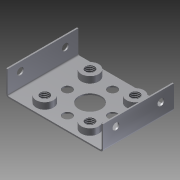
# Autodesk Inventor part: Servo Bracket
Saved by Autodesk Inventor 2012 (Build 160160000, 160)
## iProperties
Created: 2011-10-07
Part Number: Servo Bracket
Material: Default
Document SubType Name: Sheet Metal
Designer: KuttaA
Density: 1 g/cm^3
Sheet Metal Rule: Default
Author: KuttaA
Autodesk Inventor part; units mm, degrees
ref_plane "YZ Plane" through (0, 0, 0) normal (1, 0, 0) x (0, 1, 0)
ref_plane "XZ Plane" through (0, 0, 0) normal (0, 1, 0) x (-1, 0, 0)
ref_plane "XY Plane" through (0, 0, 0) normal (0, 0, 1) x (1, 0, 0)
sketch "Sketch1" plane through (0, 0, 0) normal (0, 0, 1) x (1, 0, 0)
  line L0 (-17.23, 12.6) -> (17.23, 12.6)
  line L1 (17.23, 12.6) -> (17.23, -12.6)
  line L2 (17.23, -12.6) -> (-17.23, -12.6)
  line L3 (-17.23, -12.6) -> (-17.23, 12.6)
  point P0 (0, 0)
  dimension "d0" = 17.23
  dimension "d1" = 34.46
  dimension "d2" = 12.6
  dimension "d3" = 25.2
  measures "d0" distance from line of L1 point (0, 0)
  measures "d1" distance between parallel lines of L1 L3
  measures "d2" distance from line of L0 point (0, 0)
  measures "d3" distance of L2.end L0.start
extrude "Plate1" add sketch "Sketch1" along normal blind 0.5
sketch "Sketch4" plane through (-16.73, -12.6, 0) normal (-1, 0, 0) x (0, -1, 0)
  line L0 (-25.2, 0) -> (0, 0)
  line L1 (0, 0) -> (0, 8.75)
  line L2 (0, 8.75) -> (-25.2, 8.75)
  line L3 (-25.2, 8.75) -> (-25.2, 0)
  constraints: 4 end point, 4 other
edge flange "Flange1" height 8.75 angle 90 thickness 0.5 bend radius 0.5 thickness toward (-1, 0, 0) relief tear relief width 0.5 relief depth 0.25 edges at (-17.23, 0, 0.5) wall of the first edge with corners at (-16.73, 12.6, 0) (-16.73, -12.6, 0) (-16.73, -12.6, 8.75) (-16.73, 12.6, 8.75)
bend "Bend1"
corner "Corner1"
sketch "Sketch5" plane through (16.73, 12.6, 0) normal (1, 0, 0) x (0, 1, 0)
  line L0 (-25.2, 0) -> (0, 0)
  line L1 (0, 0) -> (0, 8.75)
  line L2 (0, 8.75) -> (-25.2, 8.75)
  line L3 (-25.2, 8.75) -> (-25.2, 0)
  constraints: 4 end point, 4 other
edge flange "Flange2" height 8.75 angle 90 thickness 0.5 bend radius 0.5 thickness toward (1, 0, 0) relief tear relief width 0.5 relief depth 0.25 edges at (17.23, 0, 0.5) wall of the first edge with corners at (16.73, -12.6, 0) (16.73, 12.6, 0) (16.73, 12.6, 8.75) (16.73, -12.6, 8.75)
bend "Bend2"
corner "Corner2"
sketch "Sketch6" plane through (0, 0, 0.5) normal (0, 0, 1) x (1, 0, 0)
  circle A0 centre (0, 0) radius 4
  circle A1 centre (0, 8.04) radius 1.65
  circle A2 centre (0, -8.04) radius 1.65
  circle A3 centre (8.04, 0) radius 1.65
  circle A4 centre (-8.04, 0) radius 1.65
  line L0 (16.23, -12.6) -> (-16.23, -12.6) projected
  line L1 (-16.23, 12.6) -> (16.23, 12.6) projected
  dimension "d26" = 3.3
  dimension "d27" = 8
  dimension "d29" = 4.56
  dimension "d30" = 4.56
  dimension "d31" = 8.04
  dimension "d32" = 8.04
  dimension "d33" = 8.04
  constraints: 5 centre point, 3 equal radius, 1 coincident
  measures "d26" diameter of A4
  measures "d27" diameter of A0
  measures "d29" distance from line of L0 A2.centre
  measures "d30" distance from line of A1.centre L1
  measures "d31" distance of point (0, 0) A1.centre
  measures "d32" distance of A3.centre point (0, 0)
  measures "d33" distance of A4.centre point (0, 0)
extrude "Extrusion1" cut sketch "Sketch6" against normal through all
sketch "Sketch7" plane through (0, 0, 0.5) normal (0, 0, 1) x (1, 0, 0)
  circle A0 centre (0, 8.04) radius 1.65 projected
  circle A1 centre (-8.04, 0) radius 1.65 projected
  circle A2 centre (-8.04, 8.04) radius 1.6
  line L0 (0, -17.64) -> (0, 17.64) projected
  line L1 (-24.122, 0) -> (24.122, 0) projected
  circle A3 centre (8.04, 8.04) radius 1.6
  circle A4 centre (-8.04, -8.04) radius 1.6
  circle A5 centre (8.04, -8.04) radius 1.6
  point P0 (0, 0)
  dimension "d36" = 3.2
  constraints: 4 centre point, 3 symmetric about line, 3 other
  measures "d36" diameter of A2
extrude "Extrusion2" cut sketch "Sketch7" against normal through all contours A2 | A3 | A4 | A5
sketch "Sketch8" plane through (0, 0, 0.5) normal (0, 0, 1) x (1, 0, 0)
  circle A0 centre (-8.04, 8.04) radius 1.6 projected
  circle A1 centre (8.04, 8.04) radius 1.6 projected
  circle A2 centre (8.04, -8.04) radius 1.6 projected
  circle A3 centre (-8.04, -8.04) radius 1.6 projected
  circle A4 centre (-8.04, 8.04) radius 3.1
  circle A5 centre (8.04, 8.04) radius 3.1
  circle A6 centre (8.04, -8.04) radius 3.1
  circle A7 centre (-8.04, -8.04) radius 3.1
  point P0 (0, 0)
  dimension "d39" = 6.2
  constraints: 4 centre point, 4 coincident, 3 equal radius
  measures "d39" diameter of A4
extrude "Extrusion3" add sketch "Sketch8" along normal blind 2.28
thread "Thread1" size "M3.5x0.6" class "6H" standard "ANSI Metric M Profile" full length
thread "Thread2" size "M3.5x0.6" class "6H" standard "ANSI Metric M Profile" full length
thread "Thread3" size "M3.5x0.6" class "6H" standard "ANSI Metric M Profile" full length
thread "Thread4" size "M3.5x0.6" class "6H" standard "ANSI Metric M Profile" full length
sketch "Sketch9" plane through (-17.23, -12.6, 8.75) normal (-1, 0, 0) x (0, 0, 1)
  circle A0 centre (-3.5174, 20.57) radius 1.2
  circle A1 centre (-2.9878, 4.57) radius 1.2
  line L0 (-7.75, 25.2) -> (0, 25.2) projected
  point P0 (-8.75, 12.6)
  dimension "d50" = 2.4
  dimension "d51" = 16
  dimension "d52" = 4.63
  constraints: 2 centre point, 1 equal radius
  measures "d50" diameter of A0
  measures "d51" vertical distance of A1.centre A0.centre
  measures "d52" distance from line of L0 A0.centre
extrude "Extrusion4" cut sketch "Sketch9" against normal through all
equation "\"d30\" = d29"
equation "\"d6\" = BendReliefWidth"
equation "\"d7\" = BendReliefDepth"
equation "\"d8\" = MinimumRemnant"
equation "\"d9\" = BendRadius"
equation "\"d12\" = BendRadius"
equation "\"d13\" = CornerReliefSize"
equation "\"d14\" = GapSize"
equation "\"d15\" = JacobiRadiusSize"
equation "\"d16\" = BendReliefWidth"
equation "\"d17\" = BendReliefDepth"
equation "\"d18\" = MinimumRemnant"
equation "\"d19\" = BendRadius"
equation "\"d22\" = BendRadius"
equation "\"d23\" = CornerReliefSize"
equation "\"d24\" = GapSize"
equation "\"d25\" = JacobiRadiusSize"
equation "\"d32\" = d31"
equation "\"d33\" = d32"
equation "\"d0\" = 0.5 * d1"
equation "\"d2\" = 0.5 * d3"
equation "\"BendRadius\" = Thickness"
equation "\"BendReliefWidth\" = Thickness"
equation "\"BendReliefDepth\" = 0.5 * Thickness"
equation "\"CornerReliefSize\" = 4 * Thickness"
equation "\"MinimumRemnant\" = 2 * Thickness"
equation "\"TransitionRadius\" = BendRadius"
equation "\"JacobiRadiusSize\" = Thickness"
equation "\"GapSize\" = Thickness"
equation "\"d4\" = BendRadius"
equation "\"Thickness\" = 0.5"
body "Solid1"
